Autodesk Inventor part; units mm, degrees
(part 2 of 2)
sketch "Szkic114" plane through (0, -10, 0) normal (0, -1, 0) x (1, 0, 0)
  circle A0 centre (-56.5004, -127.7812) radius 39.5
  circle A1 centre (-37.35, -79.531) radius 1.5 projected
  circle A2 centre (-37.35, -34.531) radius 1.5 projected
  circle A3 centre (-92.2504, -163.5312) radius 2.25 projected
  circle A4 centre (-20.7504, -92.0312) radius 2.25 projected
  circle A5 centre (-20.7504, -163.5312) radius 2.25 projected
  circle A6 centre (-92.2504, -92.0312) radius 2.25 projected
  line L0 (0, -200) -> (0, 0) projected
  line L1 (0, 0) -> (-200, 0) projected
  line L2 (-185, -15) -> (-144.5, -15) projected
  line L3 (-144.5, -15) -> (-144.5, -55.5) projected
  line L4 (-144.5, -55.5) -> (-185, -55.5) projected
  line L5 (-185, -55.5) -> (-185, -15) projected
  line L6 (-200, 0) -> (-200, -200) projected
  line L7 (-185, -185) -> (-185, -144.5) projected
  line L8 (-185, -144.5) -> (-144.5, -144.5) projected
  line L9 (-144.5, -144.5) -> (-144.5, -185) projected
  line L10 (-144.5, -185) -> (-185, -185) projected
  line L11 (-200, -200) -> (0, -200) projected
  line L12 (-96.437, -60.4995) -> (-96.437, -78.1625)
  line L13 (-96.437, -78.1625) -> (-63.2932, -78.1625)
  line L14 (-63.2932, -78.1625) -> (-63.2932, -60.6808)
  line L15 (-96.437, -60.4995) -> (-96.437, -42.8365)
  line L16 (-96.437, -42.8365) -> (-63.2932, -42.8365)
  line L17 (-63.2932, -42.8365) -> (-63.2932, -60.6808)
  dimension "d560" = 79
  dimension "d565" = 17.663
  dimension "d566" = 17.663
  dimension "d567" = 33.1438
  constraints: 12 end point, 2 parallel, 1 centre point
  measures "d560" diameter of A0
  measures "d565" distance of L12.start L12.end
  measures "d566" distance of L15.start L15.end
  measures "d567" distance of L12.end L13.end
extrude "Wyciągnięcie proste95" cut sketch "Szkic114" against normal blind 10 contours A0 | L15 L16 L17 L14 L13 L12 bodies 1
fillet "Zaokrąglenie8" radius 8 4 edges at (-63.2932, -5, -78.1625) (-63.2932, -5, -42.8365) (-96.437, -5, -42.8365) (-96.437, -5, -78.1625)
sketch "Szkic120" plane through (-142.5, 0, -187) normal (0, 0, -1) x (-1, 0, 0)
  line L0 (34.5, 10.5) -> (42.5, 10.5) projected
  line L1 (34.5, 2.5) -> (34.5, 10.5) projected
  line L2 (42.5, 2.5) -> (34.5, 2.5) projected
  line L3 (42.5, 10.5) -> (42.5, 2.5) projected
  line L4 (34.5, 10.5) -> (42.5, 10.5)
  line L5 (42.5, 10.5) -> (42.5, 2.5)
  line L6 (42.5, 2.5) -> (34.5, 2.5)
  line L7 (34.5, 2.5) -> (34.5, 10.5)
  point P0 (-142.5, 0)
  constraints: 8 end point, 2 parallel, 1 horizontal, 1 perpendicular
extrude "Wyciągnięcie proste103" add sketch "Szkic120" against normal blind 2 bodies 1
sketch "Szkic121" plane through (-164.75, 100, -15) normal (0, -1, 0) x (1, 0, 0)
  line L0 (-23.2974, -158.9526) -> (-22.25, -158.9526) projected
  line L1 (-23.2974, -158.9526) -> (-22.25, -160) projected
  line L2 (-22.25, -172) -> (-22.25, -127.5) projected
  line L3 (-22.25, -172) -> (-22.25, -127.5) projected
  line L4 (-22.25, -158.9526) -> (-23.2974, -158.9526)
  line L5 (-22.25, -160) -> (-23.2974, -158.9526)
  line L6 (-22.25, -160) -> (-22.25, -158.9526)
  line L7 (-22.25, -160) -> (-22.25, -172) projected
  line L8 (-22.25, -160) -> (-22.25, -158.9526)
  point P0 (164.75, 15)
  constraints: 8 end point, 2 collinear, 1 point on line
extrude "Wyciągnięcie proste104" cut sketch "Szkic121" against normal blind 50 bodies 2
sketch "name" plane through (0, -10, 0) normal (0, -1, 0) x (1, 0, 0)
  line L0 (-144.5, -55.5) -> (-185, -55.5) projected
  line L1 (-185, -185) -> (-185, -144.5) projected
  line L2 (-81.6329, -9.0883) -> (-112.1132, -9.0883)
  line L3 (-50.7761, -9.0883) -> (-47.721, -9.0883)
  line L4 (-47.721, -9.0883) -> (-44.9414, -12.7593)
  line L5 (-44.9414, -12.7593) -> (-44.0338, -12.7593)
  line L6 (-44.0338, -12.7593) -> (-44.0338, -9.0883)
  line L7 (-44.0338, -9.0883) -> (-41.5379, -9.0883)
  line L8 (-41.5379, -9.0883) -> (-41.5379, -19.0883)
  line L9 (-41.5379, -19.0883) -> (-45.5573, -19.0883)
  spline S0 degree 2 poles (-45.5573, -19.0883) (-46.392, -19.0883) (-47.6238, -18.8776) (-48.1505, -18.5535) knots 0 0 0 1 2 2 2
  spline S1 degree 2 poles (-48.1505, -18.5535) (-48.6853, -18.2131) (-49.3174, -17.1515) (-49.3174, -16.3411) knots 0 0 0 1 2 2 2
  spline S2 degree 2 poles (-49.3174, -16.3411) (-49.3174, -15.1985) (-48.2802, -13.7642) (-47.4131, -13.3428) knots 0 0 0 1 2 2 2
  line L10 (-47.4131, -13.3428) -> (-50.7761, -9.0883)
  spline S3 degree 2 poles (-46.7405, -16.0251) (-46.7405, -16.406) (-46.4487, -16.9489) (-46.1165, -17.0948) knots 0 0 0 1 2 2 2
  spline S4 degree 2 poles (-46.1165, -17.0948) (-45.8815, -17.192) (-45.3061, -17.2488) (-44.8766, -17.2488) knots 0 0 0 1 2 2 2
  line L11 (-44.8766, -17.2488) -> (-44.0338, -17.2488)
  line L12 (-44.0338, -17.2488) -> (-44.0338, -14.5583)
  line L13 (-44.0338, -14.5583) -> (-44.755, -14.5583)
  spline S5 degree 2 poles (-44.755, -14.5583) (-45.2737, -14.5583) (-46.0111, -14.688) (-46.2623, -14.8906) knots 0 0 0 1 2 2 2
  spline S6 degree 2 poles (-46.2623, -14.8906) (-46.5054, -15.0851) (-46.7405, -15.6037) (-46.7405, -16.0251) knots 0 0 0 1 2 2 2
  line L14 (-51.5217, -9.0883) -> (-51.5217, -19.0883)
  line L15 (-51.5217, -19.0883) -> (-58.2802, -19.0883)
  line L16 (-58.2802, -19.0883) -> (-58.2802, -17.1839)
  line L17 (-58.2802, -17.1839) -> (-54.0176, -17.1839)
  line L18 (-54.0176, -17.1839) -> (-54.0176, -15.4254)
  line L19 (-54.0176, -15.4254) -> (-57.9479, -15.4254)
  line L20 (-57.9479, -15.4254) -> (-57.9479, -13.521)
  line L21 (-57.9479, -13.521) -> (-54.0176, -13.521)
  line L22 (-54.0176, -13.521) -> (-54.0176, -10.9927)
  line L23 (-54.0176, -10.9927) -> (-58.2802, -10.9927)
  line L24 (-58.2802, -10.9927) -> (-58.2802, -9.0883)
  line L25 (-58.2802, -9.0883) -> (-51.5217, -9.0883)
  line L26 (-68.3288, -19.0883) -> (-64.8928, -9.0883)
  line L27 (-64.8928, -9.0883) -> (-62.2753, -9.0883)
  line L28 (-62.2753, -9.0883) -> (-58.8393, -19.0883)
  line L29 (-58.8393, -19.0883) -> (-61.4406, -19.0883)
  line L30 (-61.4406, -19.0883) -> (-63.6205, -12.3055)
  line L31 (-63.6205, -12.3055) -> (-65.7923, -19.0883)
  line L32 (-65.7923, -19.0883) -> (-68.3288, -19.0883)
  line L33 (-72.1213, -13.9911) -> (-69.7469, -13.9911)
  line L34 (-69.7469, -13.9911) -> (-69.7469, -16.6329)
  line L35 (-69.7469, -16.6329) -> (-72.1213, -16.6329)
  line L36 (-72.1213, -16.6329) -> (-72.1213, -13.9911)
  line L37 (-72.1213, -9.0883) -> (-69.7469, -9.0883)
  line L38 (-69.7469, -9.0883) -> (-69.7469, -11.7301)
  line L39 (-69.7469, -11.7301) -> (-72.1213, -11.7301)
  line L40 (-72.1213, -11.7301) -> (-72.1213, -9.0883)
  line L41 (-85.3709, -9.0883) -> (-78.7664, -9.0883)
  line L42 (-78.7664, -9.0883) -> (-78.7664, -10.8306)
  line L43 (-78.7664, -10.8306) -> (-80.8734, -10.8306)
  line L44 (-80.8734, -10.8306) -> (-80.8734, -16.1223)
  line L45 (-80.8734, -16.1223) -> (-78.7664, -16.1223)
  line L46 (-78.7664, -16.1223) -> (-78.7664, -17.7512)
  spline S7 degree 2 poles (-78.7664, -17.7512) (-79.2283, -17.7512) (-80.144, -17.8728) (-80.4195, -18.0024) knots 0 0 0 1 2 2 2
  spline S8 degree 2 poles (-80.4195, -18.0024) (-80.7356, -18.1645) (-81.0922, -18.7074) (-81.1246, -19.1126) knots 0 0 0 1 2 2 2
  line L47 (-81.1246, -19.1126) -> (-83.3126, -19.1126)
  line L48 (-83.3126, -19.1126) -> (-83.3126, -10.8306)
  line L49 (-83.3126, -10.8306) -> (-85.3709, -10.8306)
  line L50 (-85.3709, -10.8306) -> (-85.3709, -9.0883)
  line L51 (-89.5443, -9.0883) -> (-87.17, -9.0883)
  line L52 (-87.17, -9.0883) -> (-87.17, -11.7301)
  line L53 (-87.17, -11.7301) -> (-89.5443, -11.7301)
  line L54 (-89.5443, -11.7301) -> (-89.5443, -9.0883)
  spline S9 degree 2 poles (-98.7421, -14.0883) (-98.7421, -12.7917) (-98.3288, -10.8468) (-97.8669, -10.1904) knots 0 0 0 1 2 2 2
  spline S10 degree 2 poles (-97.8669, -10.1904) (-97.4131, -9.5421) (-95.9463, -8.8776) (-94.8928, -8.8776) knots 0 0 0 1 2 2 2
  spline S11 degree 2 poles (-94.8928, -8.8776) (-93.8312, -8.8776) (-92.3725, -9.5421) (-91.9106, -10.2066) knots 0 0 0 1 2 2 2
  spline S12 degree 2 poles (-91.9106, -10.2066) (-91.4487, -10.863) (-91.0354, -12.7917) (-91.0354, -14.0883) knots 0 0 0 1 2 2 2
  spline S13 degree 2 poles (-91.0354, -14.0883) (-91.0354, -15.4173) (-91.4487, -17.2974) (-91.9187, -17.9781) knots 0 0 0 1 2 2 2
  spline S14 degree 2 poles (-91.9187, -17.9781) (-92.3888, -18.6426) (-93.8717, -19.2909) (-94.8928, -19.2909) knots 0 0 0 1 2 2 2
  spline S15 degree 2 poles (-94.8928, -19.2909) (-95.9706, -19.2909) (-97.4131, -18.6102) (-97.875, -17.9376) knots 0 0 0 1 2 2 2
  spline S16 degree 2 poles (-97.875, -17.9376) (-98.3288, -17.2812) (-98.7421, -15.3444) (-98.7421, -14.0883) knots 0 0 0 1 2 2 2
  spline S17 degree 2 poles (-96.2218, -14.0883) (-96.2218, -15.9441) (-95.614, -17.4433) (-94.8928, -17.4433) knots 0 0 0 1 2 2 2
  spline S18 degree 2 poles (-94.8928, -17.4433) (-94.1716, -17.4433) (-93.5557, -15.9441) (-93.5557, -14.0802) knots 0 0 0 1 2 2 2
  spline S19 degree 2 poles (-93.5557, -14.0802) (-93.5557, -12.2488) (-94.1716, -10.7253) (-94.8928, -10.7253) knots 0 0 0 1 2 2 2
  spline S20 degree 2 poles (-94.8928, -10.7253) (-95.6059, -10.7253) (-96.2218, -12.2488) (-96.2218, -14.0883) knots 0 0 0 1 2 2 2
  line L55 (-102.5994, -9.0883) -> (-100.2251, -9.0883)
  line L56 (-100.2251, -9.0883) -> (-100.2251, -11.7301)
  line L57 (-100.2251, -11.7301) -> (-102.5994, -11.7301)
  line L58 (-102.5994, -11.7301) -> (-102.5994, -9.0883)
  spline S21 degree 2 poles (-111.7972, -14.0883) (-111.7972, -12.7917) (-111.3839, -10.8468) (-110.922, -10.1904) knots 0 0 0 1 2 2 2
  spline S22 degree 2 poles (-110.922, -10.1904) (-110.4682, -9.5421) (-109.0014, -8.8776) (-107.9479, -8.8776) knots 0 0 0 1 2 2 2
  spline S23 degree 2 poles (-107.9479, -8.8776) (-106.8863, -8.8776) (-105.4277, -9.5421) (-104.9657, -10.2066) knots 0 0 0 1 2 2 2
  spline S24 degree 2 poles (-104.9657, -10.2066) (-104.5038, -10.863) (-104.0905, -12.7917) (-104.0905, -14.0883) knots 0 0 0 1 2 2 2
  spline S25 degree 2 poles (-104.0905, -14.0883) (-104.0905, -15.4173) (-104.5038, -17.2974) (-104.9738, -17.9781) knots 0 0 0 1 2 2 2
  spline S26 degree 2 poles (-104.9738, -17.9781) (-105.4439, -18.6426) (-106.9268, -19.2909) (-107.9479, -19.2909) knots 0 0 0 1 2 2 2
  spline S27 degree 2 poles (-107.9479, -19.2909) (-109.0257, -19.2909) (-110.4682, -18.6102) (-110.9301, -17.9376) knots 0 0 0 1 2 2 2
  spline S28 degree 2 poles (-110.9301, -17.9376) (-111.3839, -17.2812) (-111.7972, -15.3444) (-111.7972, -14.0883) knots 0 0 0 1 2 2 2
  spline S29 degree 2 poles (-109.2769, -14.0883) (-109.2769, -15.9441) (-108.6691, -17.4433) (-107.9479, -17.4433) knots 0 0 0 1 2 2 2
  spline S30 degree 2 poles (-107.9479, -17.4433) (-107.2267, -17.4433) (-106.6108, -15.9441) (-106.6108, -14.0802) knots 0 0 0 1 2 2 2
  spline S31 degree 2 poles (-106.6108, -14.0802) (-106.6108, -12.2488) (-107.2267, -10.7253) (-107.9479, -10.7253) knots 0 0 0 1 2 2 2
  spline S32 degree 2 poles (-107.9479, -10.7253) (-108.661, -10.7253) (-109.2769, -12.2488) (-109.2769, -14.0883) knots 0 0 0 1 2 2 2
  point P0 (0, 0)
  point P1 (-185, -170)
  constraints: 2 end point, 2 horizontal
extrude "Rev" cut sketch "name" against normal blind 1 bodies 1
sketch "Szkic124" plane through (0, -10, 0) normal (0, -1, 0) x (1, 0, 0)
  line L0 (0, 0) -> (-30.5, 0)
  line L1 (-30.5, 0) -> (-30.5, -15.5)
  line L2 (-30.5, -15.5) -> (0, -15.5)
  line L3 (0, -15.5) -> (0, 0)
  line L4 (0, -15.5) -> (-15.5, -15.5)
  line L5 (-15.5, -15.5) -> (-15.5, -31)
  line L6 (-15.5, -31) -> (0, -31)
  line L7 (0, -31) -> (0, -15.5)
  line L8 (-200, 0) -> (0, 0) projected
  line L9 (-100, 0) -> (-100, -5.7772)
  line L10 (0, 0) -> (0, -200) projected
  line L11 (0, -100) -> (-4.2052, -100)
  line L12 (0, -200) -> (-30.5, -200)
  line L13 (-30.5, -200) -> (-30.5, -184.5)
  line L14 (-30.5, -184.5) -> (0, -184.5)
  line L15 (0, -184.5) -> (0, -200)
  line L16 (-15.5, -184.5) -> (-15.5, -169)
  line L17 (-15.5, -169) -> (0, -169)
  line L18 (0, -169) -> (0, -184.5)
  line L19 (-144.5, -185) -> (-185, -185) projected
  line L20 (-200, -200) -> (-169.5, -200)
  line L21 (-169.5, -200) -> (-169.5, -185)
  line L22 (-169.5, -185) -> (-200, -185)
  line L23 (-200, -185) -> (-200, -200)
  line L24 (-185, -144.5) -> (-185, -185) projected
  line L25 (-200, -185) -> (-185, -185)
  line L26 (-185, -185) -> (-185, -169.5)
  line L27 (-185, -169.5) -> (-200, -169.5)
  line L28 (-200, -169.5) -> (-200, -185)
  line L29 (-144.5, -15) -> (-185, -15) projected
  line L30 (-200, 0) -> (-169.5, 0)
  line L31 (-169.5, 0) -> (-169.5, -15)
  line L32 (-169.5, -15) -> (-200, -15)
  line L33 (-200, -15) -> (-200, 0)
  line L34 (-185, -15) -> (-185, -55.5) projected
  line L35 (-200, -15) -> (-185, -15)
  line L36 (-185, -15) -> (-185, -30.5)
  line L37 (-185, -30.5) -> (-200, -30.5)
  line L38 (-200, -30.5) -> (-200, -15)
  point P0 (-185, -175)
  dimension "d604" = 30.5
  dimension "d605" = 15.5
  dimension "d606" = 15.5
  dimension "d607" = 15.5
  dimension "d610" = 30.5
  dimension "d611" = 15.5
  dimension "d612" = 30.5
  dimension "d613" = 15.5
  constraints: 66 end point, 12 parallel, 7 horizontal, 6 perpendicular, 6 symmetric about line, 4 point on line, 2 midpoint, 1 vertical
  measures "d604" distance of L2.end L1.end
  measures "d605" distance of L1.end L0.end
  measures "d606" distance of L6.end L5.end
  measures "d607" distance of L5.end L4.end
  measures "d610" distance of L22.end L21.end
  measures "d611" distance of L26.end L25.end
  measures "d612" distance of L31.end L32.end
  measures "d613" distance of L35.end L36.end
extrude "Wyciągnięcie proste107" cut sketch "Szkic124" against normal blind 2 bodies 1
sketch "Szkic125" plane through (0, -8, 0) normal (0, -1, 0) x (1, 0, 0)
  line L0 (-5.758, 0) -> (-5.758, -5.758)
  line L1 (0, 0) -> (0, -200) projected
  line L2 (0, -5.758) -> (-5.758, -5.758)
  line L3 (-30.5, 0) -> (0, 0) projected
  circle A0 centre (-5.758, -5.758) radius 1.75
  line L4 (0, -169) -> (0, -31) projected
  line L5 (-169.5, -15) -> (-169.5, 0) projected
  line L6 (-200, 0) -> (-169.5, 0) projected
  line L7 (-200, -30.5) -> (-200, 0) projected
  line L8 (-200, -169.5) -> (-200, -30.5) projected
  line L9 (-200, -200) -> (-200, -169.5) projected
  line L10 (-169.5, -200) -> (-200, -200) projected
  line L11 (-30.5, -200) -> (-169.5, -200) projected
  line L12 (0, -200) -> (-30.5, -200) projected
  line L13 (0, -169) -> (0, -200) projected
  line L14 (0, -31) -> (0, -169) projected
  line L15 (0, 0) -> (0, -31) projected
  line L16 (-30.5, 0) -> (0, 0) projected
  line L17 (-169.5, 0) -> (-30.5, 0) projected
  line L18 (-169.5, -15) -> (-185, -15) projected
  line L19 (-144.5, -15) -> (-169.5, -15) projected
  line L20 (-144.5, -55.5) -> (-144.5, -15) projected
  line L21 (-185, -55.5) -> (-144.5, -55.5) projected
  line L22 (-185, -30.5) -> (-185, -55.5) projected
  line L23 (-200, -30.5) -> (-185, -30.5) projected
  line L24 (-185, -169.5) -> (-200, -169.5) projected
  line L25 (-185, -144.5) -> (-185, -169.5) projected
  line L26 (-144.5, -144.5) -> (-185, -144.5) projected
  line L27 (-144.5, -185) -> (-144.5, -144.5) projected
  line L28 (-169.5, -185) -> (-144.5, -185) projected
  line L29 (-169.5, -200) -> (-169.5, -185) projected
  line L30 (-30.5, -184.5) -> (-30.5, -200) projected
  line L31 (-15.5, -184.5) -> (-30.5, -184.5) projected
  line L32 (-15.5, -169) -> (-15.5, -184.5) projected
  line L33 (0, -169) -> (-15.5, -169) projected
  line L34 (-15.5, -31) -> (0, -31) projected
  line L35 (-15.5, -15.5) -> (-15.5, -31) projected
  line L36 (-30.5, -15.5) -> (-15.5, -15.5) projected
  line L37 (-30.5, 0) -> (-30.5, -15.5) projected
  line L38 (-185, -15) -> (-185, -30.5) projected
  line L39 (-185, -169.5) -> (-185, -185) projected
  line L40 (-185, -185) -> (-169.5, -185) projected
  arc A1 (-63.2932, -50.8365) -> (-71.2932, -42.8365) centre (-71.2932, -50.8365) ccw projected
  line L41 (-71.2932, -42.8365) -> (-88.437, -42.8365) projected
  arc A2 (-88.437, -42.8365) -> (-96.437, -50.8365) centre (-88.437, -50.8365) ccw projected
  line L42 (-96.437, -50.8365) -> (-96.437, -70.1625) projected
  arc A3 (-96.437, -70.1625) -> (-88.437, -78.1625) centre (-88.437, -70.1625) ccw projected
  line L43 (-88.437, -78.1625) -> (-71.2932, -78.1625) projected
  arc A4 (-71.2932, -78.1625) -> (-63.2932, -70.1625) centre (-71.2932, -70.1625) ccw projected
  line L44 (-63.2932, -70.1625) -> (-63.2932, -50.8365) projected
  circle A5 centre (-56.5004, -127.7812) radius 39.5 projected
  circle A6 centre (-37.35, -79.531) radius 1.5 projected
  circle A7 centre (-37.35, -34.531) radius 1.5 projected
  circle A8 centre (-92.2504, -163.5312) radius 2.25 projected
  circle A9 centre (-20.7504, -92.0312) radius 2.25 projected
  circle A10 centre (-20.7504, -163.5312) radius 2.25 projected
  circle A11 centre (-92.2504, -92.0312) radius 2.25 projected
  line L45 (-169.5, -15) -> (-169.5, 0) projected
  line L46 (-200, 0) -> (-169.5, 0) projected
  line L47 (-200, -30.5) -> (-200, 0) projected
  line L48 (-200, -169.5) -> (-200, -30.5) projected
  line L49 (-200, -200) -> (-200, -169.5) projected
  line L50 (-169.5, -200) -> (-200, -200) projected
  line L51 (-30.5, -200) -> (-169.5, -200) projected
  line L52 (0, -200) -> (-30.5, -200) projected
  line L53 (0, -169) -> (0, -200) projected
  line L54 (0, -31) -> (0, -169) projected
  line L55 (0, 0) -> (0, -31) projected
  line L56 (-30.5, 0) -> (0, 0) projected
  line L57 (-169.5, 0) -> (-30.5, 0) projected
  line L58 (-169.5, -15) -> (-185, -15) projected
  line L59 (-144.5, -15) -> (-169.5, -15) projected
  line L60 (-144.5, -55.5) -> (-144.5, -15) projected
  line L61 (-185, -55.5) -> (-144.5, -55.5) projected
  line L62 (-185, -30.5) -> (-185, -55.5) projected
  line L63 (-200, -30.5) -> (-185, -30.5) projected
  line L64 (-185, -169.5) -> (-200, -169.5) projected
  line L65 (-185, -144.5) -> (-185, -169.5) projected
  line L66 (-144.5, -144.5) -> (-185, -144.5) projected
  line L67 (-144.5, -185) -> (-144.5, -144.5) projected
  line L68 (-169.5, -185) -> (-144.5, -185) projected
  line L69 (-169.5, -200) -> (-169.5, -185) projected
  line L70 (-30.5, -184.5) -> (-30.5, -200) projected
  line L71 (-15.5, -184.5) -> (-30.5, -184.5) projected
  line L72 (-15.5, -169) -> (-15.5, -184.5) projected
  line L73 (0, -169) -> (-15.5, -169) projected
  line L74 (-15.5, -31) -> (0, -31) projected
  line L75 (-15.5, -15.5) -> (-15.5, -31) projected
  line L76 (-30.5, -15.5) -> (-15.5, -15.5) projected
  line L77 (-30.5, 0) -> (-30.5, -15.5) projected
  line L78 (-185, -15) -> (-185, -30.5) projected
  line L79 (-185, -169.5) -> (-185, -185) projected
  line L80 (-185, -185) -> (-169.5, -185) projected
  arc A12 (-63.2932, -50.8365) -> (-71.2932, -42.8365) centre (-71.2932, -50.8365) ccw projected
  line L81 (-71.2932, -42.8365) -> (-88.437, -42.8365) projected
  arc A13 (-88.437, -42.8365) -> (-96.437, -50.8365) centre (-88.437, -50.8365) ccw projected
  line L82 (-96.437, -50.8365) -> (-96.437, -70.1625) projected
  arc A14 (-96.437, -70.1625) -> (-88.437, -78.1625) centre (-88.437, -70.1625) ccw projected
  line L83 (-88.437, -78.1625) -> (-71.2932, -78.1625) projected
  arc A15 (-71.2932, -78.1625) -> (-63.2932, -70.1625) centre (-71.2932, -70.1625) ccw projected
  line L84 (-63.2932, -70.1625) -> (-63.2932, -50.8365) projected
  circle A16 centre (-56.5004, -127.7812) radius 39.5 projected
  circle A17 centre (-37.35, -79.531) radius 1.5 projected
  circle A18 centre (-37.35, -34.531) radius 1.5 projected
  circle A19 centre (-92.2504, -163.5312) radius 2.25 projected
  circle A20 centre (-20.7504, -92.0312) radius 2.25 projected
  circle A21 centre (-20.7504, -163.5312) radius 2.25 projected
  circle A22 centre (-92.2504, -92.0312) radius 2.25 projected
  line L85 (-169.5, -200) -> (-30.5, -200) projected
  line L86 (0, -100) -> (-7.75, -100)
  circle A23 centre (-5.758, -194.242) radius 1.75
  line L87 (-30.5, 0) -> (-169.5, 0) projected
  line L88 (-100, 0) -> (-100, -5.758)
  circle A24 centre (-194.242, -5.758) radius 1.75
  circle A25 centre (-194.242, -194.242) radius 1.75
  circle A26 centre (-122.6772, -159.2778) radius 7 projected
  circle A27 centre (-122.6772, -159.2778) radius 7 projected
  dimension "d614" = 5.758
  dimension "d615" = 5.758
  dimension "d616" = 3.5
  constraints: 8 end point, 4 centre point, 3 symmetric about line, 2 horizontal, 2 midpoint, 2 point on line, 2 vertical, 1 coincident, 3 other
  measures "d614" distance of L0.start L0.end
  measures "d615" distance of L0.end L2.start
  measures "d616" diameter of A0
extrude "Wyciągnięcie proste108" cut sketch "Szkic125" against normal blind 10 contours A0 L2 L0 | L0 L2 A0 | A23 | A24 | A25 bodies 1
sketch "Szkic172" plane through (-185, 12.5, -185) normal (0, 1, 0) x (1, 0, 0)
  line L0 (0, 0) -> (0, -40.5) projected
  line L1 (8, 0) -> (8, -40.5) projected
  line L2 (0, 0) -> (8, 0)
  line L3 (8, 0) -> (8, -8)
  line L4 (8, -8) -> (0, -8)
  line L5 (0, -8) -> (0, 0)
  point P0 (185, -185)
  point P1 (0, -8)
  dimension "d1044" = 8
  constraints: 8 end point, 2 parallel, 1 horizontal, 1 perpendicular, 1 point on line
  measures "d1044" distance of L2.end L3.end
extrude "Wyciągnięcie proste109" cut sketch "Szkic172" against normal blind 2 bodies 1
sketch "Szkic173" plane through (-185, 12.5, -144.5) normal (0, 1, 0) x (1, 0, 0)
  line L0 (8, 40.5) -> (8, 32.5) projected
  line L1 (8, 32.5) -> (0, 32.5) projected
  line L2 (10, 40.5) -> (10, 0) projected
  line L3 (0, 32.5) -> (8, 32.5)
  line L4 (10, 32.5) -> (10, 30.5)
  line L5 (10, 30.5) -> (0, 30.5)
  line L6 (0, 30.5) -> (0, 32.5)
  line L7 (8, 40.5) -> (10, 40.5)
  line L8 (10, 40.5) -> (10, 32.5)
  line L9 (8, 32.5) -> (8, 40.5)
  point P0 (185, -144.5)
  constraints: 14 end point, 3 parallel, 2 horizontal, 2 perpendicular, 1 point on line
extrude "Wyciągnięcie proste110" add sketch "Szkic173" along normal blind 126 bodies 1
sketch "Szkic174" plane through (-177, 2.5, -144.5) normal (-1, 0, 0) x (0, 0, 1)
  line L0 (-30.5, 10) -> (-30.5, 97.5) projected
  line L1 (-28.5, 137.5) -> (-40.5, 137.5) projected
  line L2 (131.5, 137.5) -> (-42.5, 137.5) projected
  line L3 (-36.9776, 137.5) -> (-36.9776, 117.5)
  line L4 (-30.5, 117.5) -> (-32.5, 117.5)
  line L5 (-30.5, 10) -> (-30.5, 136) projected
  line L6 (-40.5, 97.5) -> (-40.5, 136) projected
  line L7 (-40.5, 117.5) -> (-32.5, 117.5)
  line L8 (-32.5, 117.5) -> (-32.5, 115.5)
  line L9 (-32.5, 115.5) -> (-40.5, 115.5)
  line L10 (-40.5, 115.5) -> (-40.5, 117.5)
  point P0 (144.5, -2.5)
  dimension "d1050" = 20
  dimension "d1051" = 2
  dimension "d1052" = 2
  constraints: 12 end point, 3 point on line, 2 horizontal, 2 parallel, 2 perpendicular
  measures "d1050" distance of L3.start L3.end
  measures "d1051" distance of L4.start L4.end
  measures "d1052" distance of L7.end L8.end
extrude "Wyciągnięcie proste111" cut sketch "Szkic174" against normal blind 1.4 bodies 1
sketch "Szkic175" plane through (-185, 0, -15) normal (1, 0, 0) x (0, 0, -1)
  line L0 (162, 140) -> (170, 140) projected
  line L1 (172, 140) -> (-2, 140) projected
  line L2 (165.2258, 140) -> (165.2258, 120)
  line L3 (162.3592, 120) -> (169.3592, 120)
  line L4 (169.3592, 120) -> (169.3592, 118)
  line L5 (169.3592, 118) -> (162.3592, 118)
  line L6 (162.3592, 118) -> (162.3592, 120)
  point P0 (-15, 0)
  dimension "d1055" = 20
  dimension "d1056" = 2
  dimension "d1057" = 7
  constraints: 10 end point, 2 parallel, 2 perpendicular, 1 horizontal, 1 point on line
  measures "d1055" distance of L2.start L2.end
  measures "d1056" distance of L3.end L4.end
  measures "d1057" distance of L4.end L5.end
extrude "Wyciągnięcie proste112" cut sketch "Szkic175" against normal blind 1.4 bodies 2
sketch "Szkic176" plane through (-177, 10.5, -177) normal (0, 0, -1) x (-1, 0, 0)
  line L0 (8, 129.5) -> (-4, 129.5) projected
  line L1 (10, 129.5) -> (-34.5, 129.5) projected
  line L2 (3.1875, 129.5) -> (3.1875, 94.5)
  line L3 (0.3873, 94.5) -> (7.6333, 94.5)
  line L4 (7.6333, 94.5) -> (7.6333, 92.5)
  line L5 (7.6333, 92.5) -> (0.3873, 92.5)
  line L6 (0.3873, 92.5) -> (0.3873, 94.5)
  point P0 (-177, -10.5)
  dimension "d1060" = 35
  dimension "d1061" = 2
  constraints: 10 end point, 2 parallel, 1 horizontal, 1 perpendicular, 1 point on line, 1 vertical
  measures "d1060" distance of L2.start L2.end
  measures "d1061" distance of L3.end L4.end
extrude "Wyciągnięcie proste113" cut sketch "Szkic176" against normal blind 1.4 bodies 1
sketch "Szkic177" plane through (-187, 0, -185) normal (0, 0, 1) x (1, 0, 0)
  line L0 (2, 140) -> (10, 140) projected
  line L1 (5.066, 140) -> (5.066, 105)
  line L2 (2.4525, 105) -> (9.5028, 105)
  line L3 (9.5028, 105) -> (9.5028, 103)
  line L4 (9.5028, 103) -> (2.4525, 103)
  line L5 (2.4525, 103) -> (2.4525, 105)
  point P0 (187, 0)
  dimension "d1064" = 35
  dimension "d1065" = 2
  constraints: 10 end point, 2 parallel, 1 horizontal, 1 perpendicular, 1 point on line, 1 vertical
  measures "d1064" distance of L1.start L1.end
  measures "d1065" distance of L2.end L3.end
extrude "Wyciągnięcie proste114" cut sketch "Szkic177" against normal blind 1.4 bodies 2
sketch "Szkic178" plane through (-185, 102, -55.5) normal (0, 1, 0) x (1, 0, 0)
  line L0 (0, 0) -> (0, 89) projected
  line L1 (40.5, 89) -> (0, 89)
  line L2 (0, 89) -> (0, 0)
  line L3 (0, 0) -> (40.5, 0)
  line L4 (40.5, 0) -> (40.5, 89)
  point P0 (185, -55.5)
  constraints: 8 end point, 2 parallel, 1 horizontal, 1 perpendicular
extrude "Wyciągnięcie proste115" cut sketch "Szkic178" against normal blind 2 bodies 2
sketch "Szkic179" plane through (-142.5, 100, -187) normal (1, 0, 0) x (0, 0, -1)
  line L0 (-174, 40) -> (0, 40) projected
  line L1 (-100.698, 40) -> (-100.698, 37.15)
  line L2 (-174, 0) -> (-174, 40) projected
  line L3 (-174, 37.15) -> (-100.698, 37.15)
  line L4 (-100.698, 37.15) -> (-65.298, 37.15)
  circle A0 centre (-100.698, 37.15) radius 1.25
  circle A1 centre (-65.298, 37.15) radius 1.25
  point P0 (-187, -100)
  dimension "d1070" = 2.85
  dimension "d1071" = 73.302
  dimension "d1072" = 35.4
  dimension "d1073" = 2.5
  dimension "d1074" = 2.5
  constraints: 6 end point, 4 point on line, 2 centre point, 2 coincident, 1 horizontal, 1 perpendicular, 1 vertical
  measures "d1070" distance of L1.start L1.end
  measures "d1071" distance of L3.start L3.end
  measures "d1072" distance of L3.end L4.end
  measures "d1073" diameter of A0
  measures "d1074" diameter of A1
extrude "Wyciągnięcie proste116" cut sketch "Szkic179" against normal blind 2 contours A0 L4 L1 | L1 L3 A0 | L3 L4 A0 | A1 bodies 2
sketch "Szkic180" plane through (0, 100, 0) normal (0, 1, 0) x (1, 0, 0)
  line L0 (-185, 55.5) -> (-144.5, 55.5) projected
  line L1 (-185, 55.5) -> (-185, 53.5)
  line L2 (-185, 15) -> (-185, 55.5) projected
  line L3 (-185, 57.5) -> (-185, 60.5)
  line L4 (-142.5, 57.5) -> (-187, 57.5) projected
  line L5 (-185, 55.5) -> (-185, 57.5) projected
  line L6 (-185, 59.5) -> (-185, 53.5)
  line L7 (-187, 57.5) -> (-142.5, 57.5) projected
  line L8 (-185, 60.5) -> (-144.5, 60.5)
  line L9 (-144.5, 60.5) -> (-144.5, 57.5)
  line L10 (-144.5, 57.5) -> (-185, 57.5)
  line L11 (-185, 57.5) -> (-185, 60.5)
  line L12 (-144.5, 139.5) -> (-185, 139.5)
  line L13 (-144.5, 142.5) -> (-144.5, 139.5)
  line L14 (-185, 142.5) -> (-144.5, 142.5)
  line L15 (-185, 139.5) -> (-185, 142.5)
  point P0 (0, 0)
  dimension "d1078" = 3
  dimension "d1083" = 82
  constraints: 24 end point, 2 parallel, 2 point on line, 2 vertical, 1 horizontal, 1 perpendicular, 9 other
  measures "d1078" distance of L3.start L3.end
  measures "d1083" distance of L9.end L12.start
extrude "Wyciągnięcie proste117" add sketch "Szkic180" against normal blind 10 bodies 1
sketch "Szkic181" plane through (0, 100, 0) normal (0, 1, 0) x (1, 0, 0)
  line L0 (-185, 55.5) -> (-144.5, 55.5) projected
  line L1 (-180, 55.5) -> (-180, 58)
  circle A0 centre (-180, 58) radius 1.5
  line L2 (-185, 57.5) -> (-185, 60.5) projected
  line L3 (-185, 58) -> (-180, 58)
  line L4 (-144.5, 57.5) -> (-144.5, 60.5) projected
  line L5 (-144.5, 58) -> (-149.5, 58)
  circle A1 centre (-149.5, 58) radius 1.5
  circle A2 centre (-149.5, 142) radius 1.5
  circle A3 centre (-180, 142) radius 1.5
  line L6 (-185, 57.5) -> (-144.5, 57.5) projected
  point P0 (0, 0)
  point P1 (-181.5, 58)
  point P2 (-180, 56.5)
  dimension "d1089" = 3
  dimension "d1090" = 2.5
  dimension "d1091" = 5
  dimension "d1092" = 5
  dimension "d1093" = 3
  dimension "d1096" = 84
  constraints: 6 end point, 4 centre point, 3 point on line, 2 coincident, 2 perpendicular, 1 horizontal, 1 vertical, 4 other
  measures "d1089" diameter of A0
  measures "d1090" distance of L1.start L1.end
  measures "d1091" distance of L3.start L3.end
  measures "d1092" distance of L5.start L5.end
  measures "d1093" diameter of A1
  measures "d1096" distance of A1.centre A2.centre
extrude "Wyciągnięcie proste118" cut sketch "Szkic181" against normal blind 3 contours A0 L6 L1 | L1 L6 A0 | L6 A0 L3 L1 | L1 L3 A0 L6 | L6 A1 | A1 L6 | A2 | A3 bodies 1
sketch "Szkic182" plane through (-185, 100, -55.5) normal (0, 1, 0) x (1, 0, 0)
  circle A0 centre (35.5, 2.5) radius 1.5 projected
  circle A1 centre (5, 2.5) radius 1.5 projected
  arc A2 (34.0858, 2) -> (36.9142, 2) centre (35.5, 2.5) ccw
  line L0 (0, 2) -> (42.5, 2) projected
  line L1 (36.9142, 2) -> (34.0858, 2)
  arc A3 (3.5858, 2) -> (6.4142, 2) centre (5, 2.5) ccw
  line L2 (6.4142, 2) -> (3.5858, 2)
  point P0 (185, -55.5)
  point P1 (6.4142, 2)
  point P2 (3.5858, 2)
  point P3 (36.9142, 2)
  point P4 (34.0858, 2)
  constraints: 4 end point, 4 point on circle, 4 point on line, 2 centre point, 2 coincident, 2 concentric
extrude "Wyciągnięcie proste119" cut sketch "Szkic182" against normal blind 10 contours L0 A0 | L0 A1 picked at (35.5, 1.6667) picked at (5, 1.6667) bodies 2
sketch "Szkic183" plane through (-144.5, 0, -55.5) normal (-1, 0, 0) x (0, 0, 1)
  line L0 (42.5, 140) -> (-131.5, 140) projected
  line L1 (18.7855, 140) -> (18.7855, 132)
  line L2 (1.0499, 132) -> (32.2499, 132)
  line L3 (16.6499, 132) -> (16.6499, 72.4)
  line L4 (16.6499, 72.4) -> (21.1499, 72.4)
  line L5 (21.1499, 72.4) -> (12.1499, 72.4)
  line L6 (12.1499, 72.4) -> (12.1499, 70.8)
  line L7 (12.1499, 70.8) -> (21.1499, 70.8)
  line L8 (21.1499, 70.8) -> (21.1499, 72.4)
  line L9 (32.2499, 132) -> (32.2499, 112)
  line L10 (32.2499, 112) -> (33.8499, 112)
  line L11 (33.8499, 112) -> (33.8499, 107)
  line L12 (33.8499, 107) -> (32.2499, 107)
  line L13 (32.2499, 107) -> (32.2499, 112)
  line L14 (1.0499, 111.9988) -> (-0.5501, 111.9988)
  line L15 (-0.5501, 111.9988) -> (-0.5501, 106.9989)
  line L16 (-0.5501, 106.9989) -> (1.0499, 106.9989)
  line L17 (1.0499, 106.9989) -> (1.0499, 111.9988)
  line L18 (1.0499, 132) -> (1.0499, 111.9988)
  point P0 (55.5, 0)
  dimension "d1105" = 8
  dimension "d1107" = 31.2
  dimension "d1108" = 59.6
  dimension "d1109" = 4.5
  dimension "d1110" = 9
  dimension "d1111" = 1.6
  dimension "d1112" = 20
  dimension "d1113" = 1.6
  dimension "d1114" = 5
  dimension "d1115" = 1.6
  constraints: 36 end point, 7 parallel, 5 horizontal, 3 perpendicular, 2 point on line, 2 vertical, 1 collinear, 1 midpoint
  measures "d1105" distance of L1.start L1.end
  measures "d1107" distance of L2.start L2.end
  measures "d1108" distance of L3.start L3.end
  measures "d1109" distance of L3.end L4.end
  measures "d1110" distance of L7.end L6.end
  measures "d1111" distance of L6.end L5.end
  measures "d1112" distance of L2.end L9.end
  measures "d1113" distance of L11.end L12.end
  measures "d1114" distance of L10.end L11.end
  measures "d1115" distance of L16.end L15.end
extrude "Wyciągnięcie proste120" add sketch "Szkic183" along normal blind 15.6 contours L10 L11 L12 L13 | L17 L16 L15 L14 bodies 2
sketch "Szkic184" plane through (-144.5, 0, -55.5) normal (-1, 0, 0) x (0, 0, 1)
  line L0 (0, 50) -> (7.5, 50) projected
  line L1 (7.5, 50) -> (7.5, 72.4)
  line L2 (0.177, 72.4) -> (12.327, 72.4)
  line L3 (12.327, 72.4) -> (21.327, 72.4)
  line L4 (21.327, 72.4) -> (21.327, 70.8)
  line L5 (21.327, 70.8) -> (12.327, 70.8)
  line L6 (12.327, 70.8) -> (12.327, 72.4)
  point P0 (55.5, 0)
  dimension "d1118" = 22.4
  dimension "d1119" = 12.15
  dimension "d1120" = 9
  dimension "d1121" = 1.6
  constraints: 12 end point, 2 horizontal, 2 parallel, 1 perpendicular, 1 point on line, 1 vertical
  measures "d1118" distance of L0.end L1.end
  measures "d1119" distance of L2.start L2.end
  measures "d1120" distance of L4.end L5.end
  measures "d1121" distance of L3.end L4.end
extrude "Wyciągnięcie proste121" add sketch "Szkic184" along normal blind 6.6 bodies 2
sketch "Szkic185" plane through (-144.5, 72.4, -34.173) normal (0, 1, 0) x (1, 0, 0)
  line L0 (0, 9) -> (-6.6, 9) projected
  line L1 (0, 0) -> (-6.6, 0) projected
  line L2 (-6.6, 9) -> (-5, 9)
  line L3 (-5, 9) -> (-5, 0)
  line L4 (-5, 0) -> (-6.6, 0)
  line L5 (-6.6, 0) -> (-6.6, 9)
  point P0 (144.5, -34.173)
  point P1 (-5, 9)
  dimension "d1124" = 1.6
  constraints: 8 end point, 2 parallel, 1 horizontal, 1 perpendicular, 1 point on line
  measures "d1124" distance of L3.end L4.end
extrude "Wyciągnięcie proste122" add sketch "Szkic185" along normal blind 7 bodies 2
sketch "Szkic186" plane through (-144.5, 107, -23.2501) normal (0, 0, -1) x (-1, 0, 0)
  line L0 (15.6, 0) -> (15.6, 5) projected
  line L1 (0, 0) -> (15.6, 0) projected
  line L2 (15.6, 5) -> (14, 5)
  line L3 (14, 5) -> (14, 0)
  line L4 (14, 0) -> (15.6, 0)
  line L5 (15.6, 0) -> (15.6, 5)
  point P0 (-144.5, -107)
  dimension "d1127" = 1.6
  constraints: 8 end point, 2 parallel, 1 horizontal, 1 perpendicular, 1 point on line
  measures "d1127" distance of L4.end L3.end
extrude "Wyciągnięcie proste123" add sketch "Szkic186" along normal blind 32 bodies 2
sketch "Szkic187" plane through (-144.5, -10, -144.5) normal (-1, 0, 0) x (0, 0, 1)
  line L0 (131.5, 150) -> (-42.5, 150) projected
  line L1 (-22.098, 150) -> (-22.098, 80)
  line L2 (-22.098, 80) -> (-18.298, 80)
  line L3 (-18.298, 80) -> (-25.898, 80)
  line L4 (-25.898, 80) -> (-25.898, 75.9066)
  line L5 (-25.898, 75.9066) -> (-18.298, 75.9066)
  line L6 (-18.298, 75.9066) -> (-18.298, 80)
  point P0 (144.5, 10)
  dimension "d1130" = 70
  dimension "d1131" = 3.8
  dimension "d1137" = 7.6
  constraints: 12 end point, 2 horizontal, 2 parallel, 2 perpendicular, 1 point on line
  measures "d1130" distance of L1.start L1.end
  measures "d1131" distance of L1.end L2.end
  measures "d1137" distance of L5.end L4.end
extrude "Wyciągnięcie proste124" add sketch "Szkic187" along normal blind 20 bodies 1
sketch "Szkic188" plane through (-144.5, 70, -163.398) normal (0, 1, 0) x (1, 0, 0)
  line L0 (-20, 3.2) -> (-14.5, 3.2)
  circle A0 centre (-14.5, 3.2) radius 3.4
  point P0 (144.5, -163.398)
  dimension "d1135" = 5.5
  dimension "d1136" = 6.8
  constraints: 2 end point, 1 centre point, 1 coincident, 1 horizontal
  measures "d1135" distance of L0.start L0.end
  measures "d1136" diameter of A0
extrude "Wyciągnięcie proste125" cut sketch "Szkic188" against normal blind 2 bodies 1
fillet "Zaokrąglenie9" radius 1 1 edges at (-162.4, 68, -166.598)
sketch "Szkic189" plane through (-116.8544, 0, -13) normal (0, 0, 1) x (1, 0, 0)
  line L0 (20, 0) -> (0, 0) projected
  line L1 (9.636, 0) -> (9.636, 2.413)
  line L2 (0, 0) -> (0, 100) projected
  line L3 (0, 2.413) -> (9.636, 2.413)
  circle A0 centre (9.636, 2.413) radius 1.5
  line L4 (9.636, 2.413) -> (9.636, 97.587)
  circle A1 centre (9.636, 97.587) radius 1.5
  point P0 (116.8544, 0)
  dimension "d1141" = 2.413
  dimension "d1142" = 9.636
  dimension "d1143" = 3
  dimension "d1144" = 95.174
  dimension "d1145" = 3
  constraints: 6 end point, 2 centre point, 2 coincident, 2 point on line, 2 vertical, 1 horizontal
  measures "d1141" distance of L1.start L1.end
  measures "d1142" distance of L1.end L3.start
  measures "d1143" diameter of A0
  measures "d1144" distance of L4.start L4.end
  measures "d1145" diameter of A1
extrude "Wyciągnięcie proste126" cut sketch "Szkic189" against normal blind 10 contours A0 L3 L1 | L1 L4 A0 | L3 A0 L4 | A1 bodies 1
sketch "Szkic190" plane through (0, 0, 0) normal (0, 1, 0) x (1, 0, 0)
  line L0 (-117.2076, 22.46) -> (-17.2076, 22.46)
  line L1 (-96.8544, 13) -> (-17.2076, 13)
  line L2 (-17.2076, 13) -> (-29.2071, 13)
  line L3 (-29.2071, 13) -> (-29.2071, 18)
  line L4 (-29.2071, 18) -> (-17.2076, 18)
  line L5 (-17.2076, 18) -> (-17.2076, 13)
  point P0 (0, 0)
  dimension "d1148" = 100
  dimension "d1149" = 5
  constraints: 12 end point, 3 horizontal, 2 parallel, 1 perpendicular
  measures "d1148" distance of L0.start L0.end
  measures "d1149" distance of L2.end L3.end
extrude "Wyciągnięcie proste127" add sketch "Szkic190" along normal blind 100 bodies 1
sketch "Szkic191" plane through (-29.2071, 0, -13) normal (0, 0, 1) x (1, 0, 0)
  line L0 (11.9995, 0) -> (11.9995, 100) projected
  line L1 (11.9995, 2.413) -> (3.3635, 2.413)
  line L2 (11.9995, 0) -> (0, 0) projected
  line L3 (3.3635, 0) -> (3.3635, 2.413)
  circle A0 centre (3.3635, 2.413) radius 1.5
  line L4 (3.3635, 2.413) -> (3.3635, 97.587)
  circle A1 centre (3.3635, 97.587) radius 1.5
  point P0 (29.2071, 0)
  dimension "d1152" = 8.636
  dimension "d1153" = 2.413
  dimension "d1154" = 3
  dimension "d1155" = 95.174
  dimension "d1156" = 3
  constraints: 6 end point, 2 centre point, 2 coincident, 2 point on line, 2 vertical, 1 horizontal
  measures "d1152" distance of L1.start L1.end
  measures "d1153" distance of L1.end L3.start
  measures "d1154" diameter of A0
  measures "d1155" distance of L4.start L4.end
  measures "d1156" diameter of A1
extrude "Wyciągnięcie proste128" cut sketch "Szkic191" against normal blind 10 contours A0 L3 L1 | L1 L4 A0 | A0 L4 L3 | A1 bodies 1
thread "Gwint32" size "M3x0.5" class "6H" standard "ANSI Metric M Profile" full length
thread "Gwint33" size "M3x0.5" class "6H" standard "ANSI Metric M Profile" full length
thread "Gwint34" size "M3x0.5" class "6H" standard "ANSI Metric M Profile" full length
thread "Gwint35" size "M3x0.5" class "6H" standard "ANSI Metric M Profile" full length
thread "Gwint36" size "M3x0.5" class "6H" standard "ANSI Metric M Profile" full length
thread "Gwint37" size "M3x0.5" class "6H" standard "ANSI Metric M Profile" full length
thread "Gwint38" size "M3x0.5" class "6H" standard "ANSI Metric M Profile" full length
thread "Gwint39" size "M3x0.5" class "6H" standard "ANSI Metric M Profile" full length
thread "Gwint40" size "M4x0.7" class "6H" standard "ANSI Metric M Profile" full length
thread "Gwint41" size "M4x0.7" class "6H" standard "ANSI Metric M Profile" full length
thread "Gwint42" size "M4x0.7" class "6H" standard "ANSI Metric M Profile" full length
thread "Gwint43" size "M4x0.7" class "6H" standard "ANSI Metric M Profile" full length
thread "Gwint44" size "M3x0.5" class "6H" standard "ANSI Metric M Profile" full length
thread "Gwint45" size "M3x0.5" class "6H" standard "ANSI Metric M Profile" full length
thread "Gwint46" size "M3x0.5" class "6H" standard "ANSI Metric M Profile" full length
thread "Gwint47" size "M3x0.5" class "6H" standard "ANSI Metric M Profile" full length
thread "Gwint48" size "M3x0.5" class "6H" standard "ANSI Metric M Profile" full length
thread "Gwint49" size "M3x0.5" class "6H" standard "ANSI Metric M Profile" full length
thread "Gwint50" size "M3x0.5" class "6H" standard "ANSI Metric M Profile" full length
thread "Gwint51" size "M3x0.5" class "6H" standard "ANSI Metric M Profile" full length
thread "Gwint52" size "M3x0.5" class "6H" standard "ANSI Metric M Profile" full length
thread "Gwint53" size "M4.5x0.75" class "6H" standard "ANSI Metric M Profile" full length
thread "Gwint54" size "M4.5x0.75" class "6H" standard "ANSI Metric M Profile" full length
thread "Gwint55" size "M3x0.5" class "6H" standard "ANSI Metric M Profile" full length
thread "Gwint56" size "M4.5x0.75" class "6H" standard "ANSI Metric M Profile" full length
thread "Gwint57" size "M4.5x0.75" class "6H" standard "ANSI Metric M Profile" full length
thread "Gwint58" size "M3.5x0.6" class "6H" standard "ANSI Metric M Profile" full length
thread "Gwint59" size "M3.5x0.6" class "6H" standard "ANSI Metric M Profile" full length
thread "Gwint60" size "M3.5x0.6" class "6H" standard "ANSI Metric M Profile" full length
thread "Gwint61" size "M3.5x0.6" class "6H" standard "ANSI Metric M Profile" full length
thread "Gwint62" size "M14x2" class "6H" standard "ANSI Metric M Profile" full length
thread "Gwint63" size "M3x0.5" class "6H" standard "ANSI Metric M Profile" full length
thread "Gwint64" size "M3x0.5" class "6H" standard "ANSI Metric M Profile" full length
equation "\"d637\" = 55deg"
equation "\"Szkic126_Pitch\" = 2"
equation "\"d655\" = 55deg"
equation "\"Szkic128_Pitch\" = 0.6"
equation "\"d673\" = 55deg"
equation "\"Szkic130_Pitch\" = 0.6"
equation "\"d691\" = 55deg"
equation "\"Szkic132_Pitch\" = 0.6"
equation "\"d709\" = 55deg"
equation "\"Szkic134_Pitch\" = 0.6"
equation "\"d727\" = 55deg"
equation "\"Szkic136_Pitch\" = 0.5"
equation "\"d745\" = 55deg"
equation "\"Szkic138_Pitch\" = 0.5"
equation "\"d763\" = 55deg"
equation "\"Szkic140_Pitch\" = 0.75"
equation "\"d781\" = 55deg"
equation "\"Szkic142_Pitch\" = 0.75"
equation "\"d799\" = 55deg"
equation "\"Szkic144_Pitch\" = 0.75"
equation "\"d817\" = 55deg"
equation "\"Szkic146_Pitch\" = 0.75"
equation "\"d835\" = 55deg"
equation "\"Szkic148_Pitch\" = 0.5"
equation "\"d853\" = 55deg"
equation "\"Szkic150_Pitch\" = 0.5"
equation "\"d871\" = 55deg"
equation "\"Szkic152_Pitch\" = 0.5"
equation "\"d889\" = 55deg"
equation "\"Szkic154_Pitch\" = 0.5"
equation "\"d907\" = 55deg"
equation "\"Szkic156_Pitch\" = 0.5"
equation "\"d925\" = 55deg"
equation "\"Szkic158_Pitch\" = 0.5"
equation "\"d943\" = 55deg"
equation "\"Szkic160_Pitch\" = 0.5"
equation "\"d961\" = 55deg"
equation "\"Szkic162_Pitch\" = 0.5"
equation "\"d979\" = 55deg"
equation "\"Szkic164_Pitch\" = 0.5"
equation "\"d997\" = 55deg"
equation "\"Szkic166_Pitch\" = 0.5"
equation "\"d1015\" = 55deg"
equation "\"Szkic168_Pitch\" = 0.5"
equation "\"d1033\" = 55deg"
equation "\"Szkic170_Pitch\" = 0.75"
